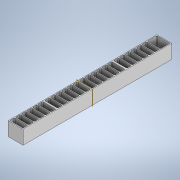
# Autodesk Inventor part: cajas
Saved by Autodesk Inventor 2020.3 (Build 243373000, 373)
## iProperties
Created: 2021-02-18
Part Number: cajas
Material: Generic
Document SubType Name: Modeling
Designer: juanp
Density: 1 g/cm^3
Appearance: Default
Author: juanp
Autodesk Inventor part; units mm, degrees
ref_plane "YZ Plane" through (0, 0, 0) normal (1, 0, 0) x (0, 1, 0)
ref_plane "XZ Plane" through (0, 0, 0) normal (0, 1, 0) x (-1, 0, 0)
ref_plane "XY Plane" through (0, 0, 0) normal (0, 0, 1) x (1, 0, 0)
sketch "Sketch1" plane through (0, 0, 0) normal (0, 1, 0) x (-1, 0, 0)
  line L0 (0, 0) -> (34, 0)
  line L1 (34, 0) -> (34, -330)
  line L2 (34, -330) -> (0, -330) construction
  line L3 (0, -330) -> (0, 0)
  line L4 (32, -2) -> (2, -2)
  line L5 (2, -2) -> (2, -12.88)
  line L6 (2, -12.88) -> (32, -12.88)
  line L7 (32, -12.88) -> (32, -2)
  line L8 (32, -14.88) -> (2, -14.88)
  line L9 (2, -14.88) -> (2, -25.76)
  line L10 (2, -25.76) -> (32, -25.76)
  line L11 (32, -25.76) -> (32, -14.88)
  line L12 (32, -27.76) -> (2, -27.76)
  line L13 (2, -27.76) -> (2, -38.64)
  line L14 (2, -38.64) -> (32, -38.64)
  line L15 (32, -38.64) -> (32, -27.76)
  line L16 (32, -40.64) -> (2, -40.64)
  line L17 (2, -40.64) -> (2, -51.52)
  line L18 (2, -51.52) -> (32, -51.52)
  line L19 (32, -51.52) -> (32, -40.64)
  line L20 (32, -53.52) -> (2, -53.52)
  line L21 (2, -53.52) -> (2, -64.4)
  line L22 (2, -64.4) -> (32, -64.4)
  line L23 (32, -64.4) -> (32, -53.52)
  line L24 (32, -66.4) -> (2, -66.4)
  line L25 (2, -66.4) -> (2, -77.28)
  line L26 (2, -77.28) -> (32, -77.28)
  line L27 (32, -77.28) -> (32, -66.4)
  line L28 (32, -81.28) -> (2, -81.28)
  line L29 (2, -81.28) -> (2, -92.16)
  line L30 (2, -92.16) -> (32, -92.16)
  line L31 (32, -92.16) -> (32, -81.28)
  line L32 (32, -94.16) -> (2, -94.16)
  line L33 (2, -94.16) -> (2, -105.04)
  line L34 (2, -105.04) -> (32, -105.04)
  line L35 (32, -105.04) -> (32, -94.16)
  line L36 (32, -107.04) -> (2, -107.04)
  line L37 (2, -107.04) -> (2, -117.92)
  line L38 (2, -117.92) -> (32, -117.92)
  line L39 (32, -117.92) -> (32, -107.04)
  line L40 (32, -119.92) -> (2, -119.92)
  line L41 (2, -119.92) -> (2, -130.8)
  line L42 (2, -130.8) -> (32, -130.8)
  line L43 (32, -130.8) -> (32, -119.92)
  line L44 (32, -132.8) -> (2, -132.8)
  line L45 (2, -132.8) -> (2, -143.68)
  line L46 (2, -143.68) -> (32, -143.68)
  line L47 (32, -143.68) -> (32, -132.8)
  line L48 (32, -145.68) -> (2, -145.68)
  line L49 (2, -145.68) -> (2, -156.56)
  line L50 (2, -156.56) -> (32, -156.56)
  line L51 (32, -156.56) -> (32, -145.68)
  line L52 (32, -160.56) -> (2, -160.56)
  line L53 (2, -160.56) -> (2, -171.44)
  line L54 (2, -171.44) -> (32, -171.44)
  line L55 (32, -171.44) -> (32, -160.56)
  line L56 (32, -173.44) -> (2, -173.44)
  line L57 (2, -173.44) -> (2, -184.32)
  line L58 (2, -184.32) -> (32, -184.32)
  line L59 (32, -184.32) -> (32, -173.44)
  line L60 (32, -186.32) -> (2, -186.32)
  line L61 (2, -186.32) -> (2, -197.2)
  line L62 (2, -197.2) -> (32, -197.2)
  line L63 (32, -197.2) -> (32, -186.32)
  line L64 (32, -199.2) -> (2, -199.2)
  line L65 (2, -199.2) -> (2, -210.08)
  line L66 (2, -210.08) -> (32, -210.08)
  line L67 (32, -210.08) -> (32, -199.2)
  line L68 (32, -212.08) -> (2, -212.08)
  line L69 (2, -212.08) -> (2, -222.96)
  line L70 (2, -222.96) -> (32, -222.96)
  line L71 (32, -222.96) -> (32, -212.08)
  line L72 (34, -330) -> (34, -340.88)
  line L73 (34, -340.88) -> (0, -340.88)
  line L74 (0, -340.88) -> (0, -330)
  line L75 (32, -224.96) -> (2, -224.96)
  line L76 (2, -224.96) -> (2, -235.84)
  line L77 (2, -235.84) -> (32, -235.84)
  line L78 (32, -235.84) -> (32, -224.96)
  line L79 (32, -239.84) -> (2, -239.84)
  line L80 (2, -239.84) -> (2, -250.72)
  line L81 (2, -250.72) -> (32, -250.72)
  line L82 (32, -250.72) -> (32, -239.84)
  line L83 (32, -252.72) -> (2, -252.72)
  line L84 (2, -252.72) -> (2, -263.6)
  line L85 (2, -263.6) -> (32, -263.6)
  line L86 (32, -263.6) -> (32, -252.72)
  line L87 (32, -265.6) -> (2, -265.6)
  line L88 (2, -265.6) -> (2, -276.48)
  line L89 (2, -276.48) -> (32, -276.48)
  line L90 (32, -276.48) -> (32, -265.6)
  line L91 (32, -278.48) -> (2, -278.48)
  line L92 (2, -278.48) -> (2, -289.36)
  line L93 (2, -289.36) -> (32, -289.36)
  line L94 (32, -289.36) -> (32, -278.48)
  line L95 (32, -291.36) -> (2, -291.36)
  line L96 (2, -291.36) -> (2, -302.24)
  line L97 (2, -302.24) -> (32, -302.24)
  line L98 (32, -302.24) -> (32, -291.36)
  line L99 (32, -304.24) -> (2, -304.24)
  line L100 (2, -304.24) -> (2, -315.12)
  line L101 (2, -315.12) -> (32, -315.12)
  line L102 (32, -315.12) -> (32, -304.24)
  line L103 (32, -317.12) -> (2, -317.12)
  line L104 (2, -317.12) -> (2, -328)
  line L105 (2, -328) -> (32, -328) construction
  line L106 (32, -328) -> (32, -317.12)
  line L107 (32, -328) -> (32, -338.88)
  line L108 (32, -338.88) -> (2, -338.88)
  line L109 (2, -338.88) -> (2, -328)
  dimension "d0" = 330
  dimension "d2" = 2
  dimension "d3" = 2
  dimension "d4" = 2
  dimension "d5" = 30
  dimension "d6" = 2
  dimension "d7" = 2
  dimension "d8" = 2
  dimension "d9" = 2
  dimension "d10" = 2
  dimension "d11" = 4
  dimension "d12" = 2
  dimension "d13" = 2
  dimension "d14" = 2
  dimension "d15" = 2
  dimension "d16" = 2
  dimension "d17" = 4
  dimension "d18" = 2
  dimension "d19" = 2
  dimension "d20" = 2
  dimension "d21" = 2
  dimension "d24" = 10.88
  dimension "d35" = 2
  dimension "d36" = 4
  dimension "d37" = 2
  dimension "d38" = 2
  dimension "d39" = 2
  dimension "d40" = 2
  dimension "d41" = 2
  dimension "d42" = 2
  dimension "d43" = 2
  dimension "d44" = 2
  constraints: 220 end point, 88 equal length, 32 point on line, 29 perpendicular, 26 horizontal, 6 collinear, 2 vertical
  measures "d0" distance of L0.end L1.end
  measures "d2" distance between parallel lines of L1 L7
  measures "d3" distance between parallel lines of L0 L4
  measures "d4" distance between parallel lines of L5 L3
  measures "d5" distance of L4.start L4.end
  measures "d6" distance between parallel lines of L8 L6
  measures "d7" distance between parallel lines of L12 L10
  measures "d8" distance between parallel lines of L16 L14
  measures "d9" distance between parallel lines of L20 L18
  measures "d10" distance between parallel lines of L22 L24
  measures "d11" distance between parallel lines of L28 L26
  measures "d12" distance between parallel lines of L32 L30
  measures "d13" distance between parallel lines of L36 L34
  measures "d14" distance between parallel lines of L40 L38
  measures "d15" distance between parallel lines of L44 L42
  measures "d16" distance between parallel lines of L48 L46
  measures "d17" distance between parallel lines of L52 L50
  measures "d18" distance between parallel lines of L56 L54
  measures "d19" distance between parallel lines of L60 L58
  measures "d20" distance between parallel lines of L64 L62
  measures "d21" distance between parallel lines of L68 L66
  measures "d24" distance of L62.end L60.start
  measures "d35" distance between parallel lines of L70 L75
  measures "d36" distance between parallel lines of L79 L77
  measures "d37" distance between parallel lines of L83 L81
  measures "d38" distance between parallel lines of L87 L85
  measures "d39" distance between parallel lines of L91 L89
  measures "d40" distance between parallel lines of L95 L93
  measures "d41" distance between parallel lines of L99 L97
  measures "d42" distance between parallel lines of L103 L101
  measures "d43" distance between parallel lines of L2 L105
  measures "d44" distance between parallel lines of L73 L108
extrude "Extrusion1" add sketch "Sketch1" along normal blind 30
sketch "Sketch3" plane through (0, 0, 0) normal (0, -1, 0) x (1, 0, 0)
  line L0 (0, 0) -> (0, -340.88) projected
  line L1 (-34, 0) -> (0, 0) projected
  line L2 (-34, -340.88) -> (-34, 0) projected
  line L3 (0, -340.88) -> (-34, -340.88) projected
extrude "Extrusion3" add sketch "Sketch3" along normal blind 2
fillet "Fillet2" radius 2 200 edges at (-32, 0, -283.92) (-2, 0, -283.92) (-32, 15, -278.48) (-17, 0, -278.48) (-32, 15, -289.36) (-17, 0, -289.36) (-17, 0, -276.48) (-32, 15, -291.36) (-2, 0, -271.04) (-17, 0, -265.6) (-2, 15, -291.36) (-2, 15, -289.36) (-2, 15, -278.48) (-2, 15, -276.48) (-2, 15, -265.6) (-32, 15, -276.48) (-32, 0, -271.04) (-17, 0, -291.36) (-32, 15, -302.24) (-32, 0, -296.8) (-2, 15, -304.24) (-32, 15, -304.24) (-32, 0, -309.68) (-17, 0, -315.12) (-2, 0, -309.68) (-17, 0, -304.24) (-32, 15, -315.12) (-2, 15, -317.12) (-32, 15, -317.12) (-17, 0, -317.12) (-2, 0, -328) (-2, 15, -338.88) (-32, 15, -338.88) (-2, 15, -315.12) (-2, 15, -302.24) (-2, 0, -296.8) (-17, 0, -302.24) (-17, 0, -338.88) (-32, 0, -328) (-2, 15, -132.8) (-2, 15, -130.8) (-2, 15, -143.68) (-2, 15, -160.56) (-2, 15, -145.68) (-32, 15, -130.8) (-32, 15, -132.8) (-2, 15, -156.56) (-32, 15, -143.68) (-32, 15, -145.68) (-32, 15, -156.56) (-32, 15, -160.56) (-32, 0, -112.48) (-17, 0, -156.56) (-32, 0, -151.12) (-2, 0, -151.12) (-17, 0, -145.68) (-17, 0, -143.68) (-32, 0, -138.24) (-2, 0, -138.24) (-17, 0, -132.8) (-17, 0, -130.8) (-32, 0, -125.36) (-2, 0, -125.36) (-17, 0, -117.92) (-2, 0, -112.48) (-17, 0, -119.92) (-17, 0, -107.04) (-32, 15, -117.92) (-2, 15, -117.92) (-2, 15, -107.04) (-32, 15, -107.04) (-32, 15, -105.04) (-2, 15, -105.04) (-2, 15, -119.92) (-32, 15, -119.92) (-2, 15, -94.16) (-32, 15, -94.16) (-32, 15, -92.16) (-2, 15, -92.16) (-2, 15, -81.28) (-32, 15, -81.28) (-32, 15, -77.28) (-2, 15, -77.28) (-2, 15, -66.4) (-32, 15, -66.4) (-32, 15, -64.4) (-2, 15, -64.4) (-32, 0, -58.96) (-17, 0, -64.4) (-17, 0, -105.04) (-32, 0, -99.6) (-2, 0, -99.6) (-17, 0, -94.16) (-17, 0, -92.16) (-32, 0, -86.72) (-2, 0, -86.72) (-17, 0, -81.28) (-32, 0, -71.84) (-2, 0, -71.84) (-17, 0, -66.4) (-2, 0, -58.96) (-17, 0, -53.52) (-17, 0, -77.28) (-2, 15, -53.52) (-32, 15, -53.52) (-32, 15, -51.52) (-2, 15, -51.52) (-2, 15, -40.64) (-32, 15, -40.64) (-32, 15, -38.64) (-2, 15, -38.64) (-2, 15, -27.76) (-32, 15, -27.76) (-32, 15, -25.76) (-2, 15, -25.76) (-2, 15, -14.88) (-32, 15, -14.88) (-32, 15, -12.88) (-32, 15, -2) (-2, 15, -2) (-2, 15, -12.88) (-32, 0, -7.44) (-17, 0, -12.88) (-17, 0, -51.52) (-32, 0, -46.08) (-2, 0, -46.08) (-17, 0, -40.64) (-17, 0, -38.64) (-32, 0, -33.2) (-2, 0, -33.2) (-17, 0, -27.76) (-17, 0, -25.76) (-32, 0, -20.32) (-17, 0, -14.88) (-17, 0, -2) (-2, 0, -7.44) (-2, 0, -20.32) (-17, 0, -160.56) (-32, 15, -252.72) (-32, 15, -239.84) (-32, 15, -263.6) (-32, 15, -265.6) (-2, 15, -250.72) (-2, 15, -252.72) (-17, 0, -252.72) (-2, 15, -239.84) (-17, 0, -239.84) (-2, 15, -263.6) (-17, 0, -263.6) (-2, 15, -235.84) (-2, 0, -230.4) (-2, 15, -224.96) (-32, 15, -250.72) (-32, 0, -258.16) (-17, 0, -250.72) (-2, 0, -245.28) (-32, 0, -245.28) (-2, 0, -258.16) (-17, 0, -235.84) (-32, 0, -230.4) (-32, 15, -235.84) (-2, 0, -217.52) (-17, 0, -224.96) (-17, 0, -222.96) (-32, 15, -224.96) (-32, 15, -222.96) (-2, 15, -222.96) (-32, 0, -217.52) (-2, 15, -212.08) (-32, 15, -212.08) (-32, 15, -210.08) (-2, 15, -210.08) (-32, 15, -199.2) (-32, 15, -197.2) (-32, 15, -186.32) (-2, 15, -186.32) (-2, 15, -197.2) (-32, 0, -166) (-17, 0, -171.44) (-17, 0, -212.08) (-17, 0, -210.08) (-2, 0, -204.64) (-32, 0, -204.64) (-17, 0, -199.2) (-17, 0, -197.2) (-2, 0, -191.76) (-32, 0, -191.76) (-17, 0, -186.32) (-17, 0, -184.32) (-17, 0, -173.44) (-32, 0, -178.88) (-2, 0, -178.88) (-2, 0, -166) (-2, 15, -184.32) (-2, 15, -173.44) (-32, 15, -173.44) (-32, 15, -171.44) (-2, 15, -171.44) (-32, 15, -184.32) (-2, 15, -199.2)
ref_plane "Work Plane1" through (-30, 30, -158.56) normal (0, 0, 1) x (1, 0, 0)
split body "Split2" result two bodies by plane through (-30, 30, -158.56) normal (0, 0, 1) first body at (-22.6667, -1.5, -105.7067)
equation "\"d2\" = grosor_pared"
equation "\"d3\" = grosor_pared"
equation "\"d4\" = grosor_pared"
equation "\"d5\" = largo_cajas"
equation "\"d6\" = grosor_pared"
equation "\"d7\" = grosor_pared"
equation "\"d8\" = grosor_pared"
equation "\"d10\" = grosor_pared"
equation "\"d12\" = grosor_pared"
equation "\"d14\" = grosor_pared"
equation "\"d15\" = grosor_pared"
equation "\"d16\" = grosor_pared"
equation "\"d17\" = 2 * grosor_pared"
equation "\"d18\" = grosor_pared"
equation "\"d19\" = grosor_pared"
equation "\"d20\" = grosor_pared"
equation "\"d21\" = grosor_pared"
equation "\"d25\" = altura_cajas"
equation "\"d32\" = grosor_pared"
equation "\"largo_cajas\" = 30"
equation "\"grosor_pared\" = 2"
equation "\"altura_cajas\" = 30"
body "Solid5"
body "Solid6"
